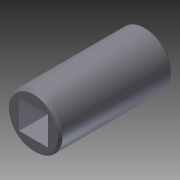
# Autodesk Inventor part: Vex Shaft Coupler
Saved by Autodesk Inventor 2014 SP1 (Build 180222100, 222)
## iProperties
Created: 2012-03-30
Part Number: Vex Shaft Coupler
Material: Steel
Document SubType Name: Modeling
Designer: Moses
Mass: 2.03148 g
Surface Area: 4.13064 cm^2
Volume: 0.258787 cm^3
Density: 7.85 g/cm^3
Appearance: Steel
Author: Moses
Autodesk Inventor part; units mm, degrees
ref_plane "YZ Plane" through (0, 0, 0) normal (1, 0, 0) x (0, 1, 0)
ref_plane "XZ Plane" through (0, 0, 0) normal (0, 1, 0) x (-1, 0, 0)
sketch "Sketch1" plane through (0, 0, 0) normal (0, 0, 1) x (1, 0, 0)
  circle A0 centre (0, 0) radius 3
  line L0 (-1.6129, 1.6129) -> (1.6129, 1.6129)
  line L1 (1.6129, 1.6129) -> (1.6129, -1.6129)
  line L2 (1.6129, -1.6129) -> (-1.6129, -1.6129)
  line L3 (-1.6129, -1.6129) -> (-1.6129, 1.6129)
  dimension "d0" = 6
  dimension "d1" = 3.2258
  dimension "d2" = 3.2258
  dimension "d3" = 1.6129
  dimension "d4" = 1.6129
  constraints: 8 end point, 2 parallel, 1 centre point, 1 coincident, 1 horizontal, 1 perpendicular
  measures "d0" diameter of A0
  measures "d1" distance of L0.start L0.end
  measures "d2" distance of L0.end L1.end
  measures "d3" distance from line of L0 point (0, 0)
  measures "d4" distance from line of L1 point (0, 0)
extrude "Extrusion1" add sketch "Sketch1" along normal blind 12.7
ref_plane "Work Plane1" through (0, 0, 6.35) normal (0, 0, 1) x (1, 0, 0)
sketch "Sketch2" plane through (0, 0, 6.35) normal (0, 0, 1) x (1, 0, 0)
  circle A0 centre (0, 0) radius 3 projected
extrude "Extrusion2" add sketch "Sketch2" along normal mid plane 3.175
chamfer "Chamfer1" distance 0.254 angle 45 2 edges at (-3, 0, 0) (-3, 0, 12.7)
equation "\"d3\" = 0.5 * d2"
equation "\"d4\" = 0.5 * d1"
body "Solid1"
